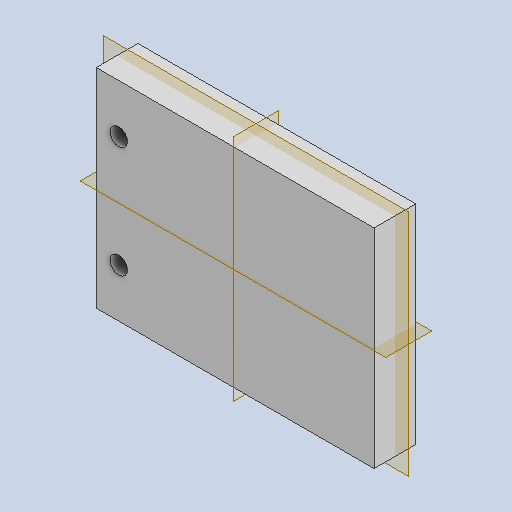
# Autodesk Inventor part: крыло
Saved by Autodesk Inventor 2023.2 (Build 272271030, 271C)
## iProperties
Created: 2024-03-20
Part Number: крыло
Material: Типовые
Document SubType Name: Modeling
Designer: I9232
Density: 1 g/cm^3
Appearance: По умолчанию
Author: I9232
Autodesk Inventor part; units mm, degrees
sketch "Эскиз1" plane through (0, 0, 0) normal (0, 0, 1) x (1, 0, 0)
  line L0 (-20, -15) -> (20, -15)
  line L1 (20, -15) -> (20, 15)
  line L2 (20, 15) -> (-20, 15)
  line L3 (-20, 15) -> (-20, -15)
  line L4 (-20, -15) -> (20, 15) construction
  line L5 (20, -15) -> (-20, 15) construction
  point P0 (0, 0)
  dimension "d0" = 40
  dimension "d1" = 30
  constraints: 12 end point, 2 midpoint, 2 parallel, 1 horizontal, 1 perpendicular
  measures "d0" distance of L1.end L2.end
  measures "d1" distance of L0.end L1.end
extrude "Выдавливание1" add sketch "Эскиз1" along normal mid plane 6
sketch "Эскиз2" plane through (0, 0, -3) normal (0, 0, -1) x (-1, 0, 0)
  circle A0 centre (16.75, 8) radius 1.25 projected
  circle A1 centre (16.75, -8) radius 1.25 projected
  point P0 (0, 0)
extrude "Выдавливание2" cut sketch "Эскиз2" against normal up to surface (6 mm away)
